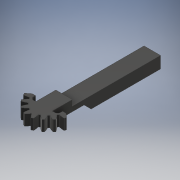
# Autodesk Inventor part: WA04
Saved by Autodesk Inventor 2017 (Build 210142000, 142)
## iProperties
Created: 2019-05-07
Part Number: WA04
Material: ABS Plastic
Document SubType Name: Modeling
Designer: Dell
Density: 1.06 g/cm^3
Appearance: Smooth - Black
Author: Dell
Autodesk Inventor part; units mm, degrees
ref_plane "YZ Plane" through (0, 0, 0) normal (1, 0, 0) x (0, 1, 0)
ref_plane "XZ Plane" through (0, 0, 0) normal (0, 1, 0) x (-1, 0, 0)
ref_plane "XY Plane" through (0, 0, 0) normal (0, 0, 1) x (1, 0, 0)
sketch "Sketch1" plane through (0, 0, 0) normal (0, 0, 1) x (1, 0, 0)
  line L0 (0, 0) -> (14, 0)
  line L1 (14, 0) -> (14, 100)
  line L2 (14, 100) -> (0, 100)
  line L3 (0, 100) -> (0, 0)
  dimension "d0" = 14
  dimension "d1" = 100
  constraints: 8 end point, 2 parallel, 1 horizontal, 1 perpendicular
  measures "d0" distance of L2.end L1.end
  measures "d1" distance of L1.end L0.end
extrude "Extrusion1" add sketch "Sketch1" along normal blind 10
sketch "Sketch2" plane through (0, 0, 10) normal (0, 0, 1) x (1, 0, 0)
  arc A0 (-7.2229, 7.2229) -> (-10.9281, 4.2365) centre (2.4249, -8.5384) ccw
  arc A1 (-10.9281, 4.2365) -> (-10.2545, 2.6798) centre (14.1758, 14.1758) ccw
  arc A2 (-10.2545, 2.6798) -> (-5.5411, 3.3364) centre (-10.4262, 21.1587) ccw
  arc A3 (-5.5411, 3.3364) -> (-4.8216, 2.1197) centre (14.1758, 14.1758) ccw
  arc A4 (-4.8216, 2.1197) -> (-7.6676, -1.6944) centre (8.4429, -10.7471) ccw
  arc A5 (-7.6676, -1.6944) -> (-6.628, -3.0346) centre (14.1758, 14.1758) ccw
  arc A6 (-6.628, -3.0346) -> (-2.226, -1.2265) centre (-11.3898, 14.8211) ccw
  arc A7 (-2.226, -1.2265) -> (-1.2265, -2.226) centre (14.1758, 14.1758) ccw
  arc A8 (-1.2265, -2.226) -> (-3.0346, -6.628) centre (14.8211, -11.3898) ccw
  arc A9 (-3.0346, -6.628) -> (-1.6944, -7.6676) centre (14.1758, 14.1758) ccw
  arc A10 (-1.6944, -7.6676) -> (2.1197, -4.8216) centre (-10.7471, 8.4429) ccw
  arc A11 (2.1197, -4.8216) -> (3.3364, -5.5411) centre (14.1758, 14.1758) ccw
  arc A12 (3.3364, -5.5411) -> (2.6798, -10.2545) centre (21.1587, -10.4262) ccw
  arc A13 (2.6798, -10.2545) -> (4.2365, -10.9281) centre (14.1758, 14.1758) ccw
  arc A14 (4.2365, -10.9281) -> (7.2229, -7.2229) centre (-8.5384, 2.4249) ccw
  circle A15 centre (14.1758, 14.1758) radius 22.5 construction
  circle A16 centre (14.1758, 14.1758) radius 27 construction
  line L0 (-7.2229, 7.2229) -> (7.2229, -7.2229)
  line L1 (-10.9281, 4.2365) -> (4.2365, -10.9281) construction
  line L2 (-5.5411, 3.3364) -> (3.3364, -5.5411) construction
  line L3 (-4.8216, 2.1197) -> (2.1197, -4.8216) construction
  line L4 (-10.2545, 2.6798) -> (2.6798, -10.2545) construction
  line L5 (-7.6676, -1.6944) -> (-1.6944, -7.6676) construction
  line L6 (-6.628, -3.0346) -> (-3.0346, -6.628) construction
  line L7 (-2.226, -1.2265) -> (-1.2265, -2.226) construction
  line L8 (0, 100) -> (0, 0) projected
  point P0 (-11.0317, -23.0721)
  point P1 (-4.9473, -25.0907)
  point P2 (1.448, -25.5328)
  point P3 (-1.448, -25.5328)
  point P4 (4.9473, -25.0907)
  point P5 (11.0317, -23.0721)
  point P6 (-1.3509, -1.3509)
  dimension "d4" = 18.4797
  dimension "d5" = 18.4797
  dimension "d6" = 27
  dimension "d7" = 27
  dimension "d8" = 27
  dimension "d9" = 27
  dimension "d10" = 18.4797
  dimension "d11" = 18.4797
  dimension "d12" = 22.5
  dimension "d13" = 22.5
  dimension "d14" = 22.5
  dimension "d15" = 18.4797
  dimension "d16" = 18.4797
  dimension "d17" = 18.4797
  dimension "d18" = 18.4797
  dimension "d19" = 4.7589
  dimension "d20" = 20.4296
  dimension "d21" = 21.446
  dimension "d22" = 9.8164
  dimension "d23" = 12.5546
  dimension "d24" = 18.2919
  dimension "d25" = 8.4475
  dimension "d26" = 5.0819
  dimension "d27" = 1.4135
  dimension "d28" = 1.559
  dimension "d31" = 45
  constraints: 30 point on circle, 16 end point, 15 centre point, 6 parallel, 2 coincident, 2 midpoint, 20 other
  measures "d4" radius of A0
  measures "d5" radius of A2
  measures "d6" radius of A1
  measures "d7" radius of A5
  measures "d8" radius of A9
  measures "d9" radius of A13
  measures "d10" radius of A12
  measures "d11" radius of A14
  measures "d12" radius of A11
  measures "d13" radius of A7
  measures "d14" radius of A3
  measures "d15" radius of A4
  measures "d16" radius of A6
  measures "d17" radius of A8
  measures "d18" radius of A10
  measures "d19" distance of L2.start L4.start
  measures "d20" distance of L0.start L0.end
  measures "d21" distance of L1.start L1.end
  measures "d22" distance of L3.start L3.end
  measures "d23" distance of L2.start L2.end
  measures "d24" distance of L4.start L4.end
  measures "d25" distance of L5.start L5.end
  measures "d26" distance of L6.start L6.end
  measures "d27" distance of L7.start L7.end
  measures "d28" distance between parallel lines of L0 L2
  measures "d31" angle of L8 L0
extrude "Extrusion2" add sketch "Sketch2" against normal blind 10
ref_plane "Work Plane1" through (7, 100, 0) normal (-1, 0, 0) x (0, 0, 1)
sketch "Sketch6" plane through (0, 0, 10) normal (0, 0, 1) x (1, 0, 0)
  circle A0 centre (7, 15) radius 2.5
  line L0 (14, 100) -> (0, 100) projected
  point P0 (0, 0)
  point P1 (7, 100)
  dimension "d38" = 5
  dimension "d39" = 85
  constraints: 1 centre point, 1 midpoint, 1 vertical alignment
  measures "d38" diameter of A0
  measures "d39" distance from line of L0 A0.centre
extrude "Extrusion6" cut sketch "Sketch6" against normal blind 10
sketch "Sketch7" plane through (0, 0, 0) normal (0, 0, -1) x (-1, 0, 0)
  circle A0 centre (-7, 14) radius 2
  circle A1 centre (-7, 15) radius 2.5 projected
  point P0 (0, 0)
  dimension "d42" = 4
  dimension "d43" = 1
  constraints: 1 centre point, 1 vertical alignment
  measures "d42" diameter of A0
  measures "d43" distance of A1.centre A0.centre
extrude "Extrusion7" add sketch "Sketch7" along normal blind 2 contours A0 A1 | A1 A0 picked at (-6.9413, 13.6767) picked at (-7.0758, 12.3503)
fillet "Fillet1" radius 2 1 edges at (9, 14, -2)
sketch "Sketch9" plane through (0, 0, 10) normal (0, 0, 1) x (1, 0, 0)
  circle A0 centre (7, 15) radius 2.5 projected
  point P0 (0, 0)
extrude "Extrusion9" add sketch "Sketch9" against normal blind 10
mirror "Mirror3" about plane through (7, 100, 0) normal (-1, 0, 0) of "Extrusion2"
sketch "Sketch10" plane through (0, 0, 0) normal (0, 0, -1) x (-1, 0, 0)
  line L0 (-14, 0) -> (-7, -7) projected
  line L1 (0, 0) -> (-14, 0) projected
  line L2 (0, 0) -> (-7, -7) projected
extrude "Extrusion10" add sketch "Sketch10" against normal blind 10
sketch "Sketch11" plane through (0, 0, 0) normal (0, 0, -1) x (-1, 0, 0)
  line L0 (-17, 3) -> (-14, 3)
  line L1 (-14, 0) -> (-14, 100) projected
  line L2 (-14, 3) -> (-14, 0)
  line L3 (-21.2229, 7.2229) -> (-14, 0) projected
  line L4 (-17, 3) -> (-14, 0)
  line L5 (0, 0) -> (0, 3)
  line L6 (0, 100) -> (0, 0) projected
  line L7 (0, 3) -> (3, 3)
  line L8 (7.2229, 7.2229) -> (0, 0) projected
  line L9 (3, 3) -> (0, 0)
  dimension "d55" = 3
  constraints: 12 end point, 3 collinear, 3 point on line, 1 horizontal, 1 horizontal alignment, 1 perpendicular
  measures "d55" distance from line of L1.start L0
extrude "Extrusion11" add sketch "Sketch11" against normal blind 10
sketch "Sketch12" plane through (0, 0, 0) normal (0, 0, -1) x (-1, 0, 0)
  line L0 (-21.2229, 7.2229) -> (-18.5, 7.2229)
  line L1 (-18.5, 7.2229) -> (-18.5, 4.5)
  line L2 (-21.2229, 7.2229) -> (-17, 3) projected
  point P0 (0, 0)
  dimension "d58" = 1.5
  constraints: 4 end point, 1 horizontal, 1 point on line, 1 vertical
  measures "d58" horizontal distance of L2.end L1.end
extrude "Extrusion12" add sketch "Sketch12" against normal blind 10
mirror "Mirror4" about plane through (7, 100, 0) normal (-1, 0, 0) of "Extrusion12"
fillet "Fillet2" radius 2 2 edges at (18.5, 4.5, 5) (-4.5, 4.5, 5)
fillet "Fillet3" radius 2 2 edges at (17, 3, 5) (-3, 3, 5)
sketch "Sketch13" plane through (0, 0, 0) normal (0, 0, -1) x (-1, 0, 0)
  line L0 (-14, 3) -> (-14, 100) projected
  line L1 (0, 100) -> (0, 3) projected
  line L2 (-14, 100) -> (0, 100)
  line L3 (0, 100) -> (0, 20)
  line L4 (0, 20) -> (-14, 20)
  line L5 (-14, 20) -> (-14, 100)
  point P0 (0, 0)
  dimension "d63" = 80
  constraints: 8 end point, 2 parallel, 1 horizontal, 1 perpendicular, 1 point on line
  measures "d63" distance between parallel lines of L2 L4
extrude "Extrusion13" cut sketch "Sketch13" against normal through all
sketch "Sketch15" plane through (14, 3, 10) normal (1, 0, 0) x (0, 0, -1)
  line L0 (0, 17) -> (10, 17) projected
  line L1 (6, 17) -> (6, 92)
  line L2 (6, 92) -> (16, 92)
  line L3 (16, 92) -> (16, 27)
  line L4 (10, 17) -> (6, 17)
  line L5 (10, 0) -> (10, 17) projected
  line L6 (10, 17) -> (0, 17) projected
  line L7 (10, 17) -> (10, 27)
  line L8 (10, 27) -> (16, 27)
  point P0 (10, -3)
  dimension "d74" = 6
  dimension "d75" = 10
  dimension "d76" = 75
  dimension "d80" = 10
  constraints: 12 end point, 4 perpendicular, 2 vertical, 1 point on line
  measures "d74" distance from line of L0.start L1
  measures "d75" distance between parallel lines of L3 L1
  measures "d76" distance between parallel lines of L0 L2
  measures "d80" distance of L0.end L7.end
extrude "Extrusion15" add sketch "Sketch15" against normal blind 14
chamfer "Chamfer1" distance 6 angle 45 1 edges at (7, 30, -6)
sketch "Sketch16" plane through (0, 0, 10) normal (0, 0, 1) x (1, 0, 0)
  circle A0 centre (7, 14) radius 2 projected
  line L0 (14, 20) -> (0, 20) projected
  line L1 (0, 20) -> (0, 3) projected
  line L2 (0, 3) -> (-2.1716, 3) projected
  arc A1 (-3.5858, 3.5858) -> (-2.1716, 3) centre (-2.1716, 5) ccw projected
  line L3 (-3.9142, 3.9142) -> (-3.5858, 3.5858) projected
  arc A2 (-4.5, 5.3284) -> (-3.9142, 3.9142) centre (-2.5, 5.3284) ccw projected
  line L4 (-4.5, 7.2229) -> (-4.5, 5.3284) projected
  line L5 (-7.2229, 7.2229) -> (-4.5, 7.2229) projected
  arc A3 (-7.2229, 7.2229) -> (-10.9281, 4.2365) centre (2.4249, -8.5384) ccw projected
  arc A4 (-10.9281, 4.2365) -> (-10.2545, 2.6798) centre (14.1758, 14.1758) ccw projected
  arc A5 (-10.2545, 2.6798) -> (-5.5411, 3.3364) centre (-10.4262, 21.1587) ccw projected
  arc A6 (-5.5411, 3.3364) -> (-4.8216, 2.1197) centre (14.1758, 14.1758) ccw projected
  arc A7 (-4.8216, 2.1197) -> (-7.6676, -1.6944) centre (8.4429, -10.7471) ccw projected
  arc A8 (-7.6676, -1.6944) -> (-6.628, -3.0346) centre (14.1758, 14.1758) ccw projected
  arc A9 (-6.628, -3.0346) -> (-2.226, -1.2265) centre (-11.3898, 14.8211) ccw projected
  arc A10 (-2.226, -1.2265) -> (-1.2265, -2.226) centre (14.1758, 14.1758) ccw projected
  arc A11 (-1.2265, -2.226) -> (-3.0346, -6.628) centre (14.8211, -11.3898) ccw projected
  arc A12 (-3.0346, -6.628) -> (-1.6944, -7.6676) centre (14.1758, 14.1758) ccw projected
  arc A13 (-1.6944, -7.6676) -> (2.1197, -4.8216) centre (-10.7471, 8.4429) ccw projected
  arc A14 (2.1197, -4.8216) -> (3.3364, -5.5411) centre (14.1758, 14.1758) ccw projected
  arc A15 (3.3364, -5.5411) -> (2.6798, -10.2545) centre (21.1587, -10.4262) ccw projected
  arc A16 (2.6798, -10.2545) -> (4.2365, -10.9281) centre (14.1758, 14.1758) ccw projected
  arc A17 (4.2365, -10.9281) -> (7, -7.578) centre (-8.5384, 2.4249) ccw projected
  arc A18 (7, -7.578) -> (9.7635, -10.9281) centre (22.5384, 2.4249) ccw projected
  arc A19 (9.7635, -10.9281) -> (11.3202, -10.2545) centre (-0.1758, 14.1758) ccw projected
  arc A20 (11.3202, -10.2545) -> (10.6636, -5.5411) centre (-7.1587, -10.4262) ccw projected
  arc A21 (10.6636, -5.5411) -> (11.8803, -4.8216) centre (-0.1758, 14.1758) ccw projected
  arc A22 (11.8803, -4.8216) -> (15.6944, -7.6676) centre (24.7471, 8.4429) ccw projected
  arc A23 (15.6944, -7.6676) -> (17.0346, -6.628) centre (-0.1758, 14.1758) ccw projected
  arc A24 (17.0346, -6.628) -> (15.2265, -2.226) centre (-0.8211, -11.3898) ccw projected
  arc A25 (15.2265, -2.226) -> (16.226, -1.2265) centre (-0.1758, 14.1758) ccw projected
  arc A26 (16.226, -1.2265) -> (20.628, -3.0346) centre (25.3898, 14.8211) ccw projected
  arc A27 (20.628, -3.0346) -> (21.6676, -1.6944) centre (-0.1758, 14.1758) ccw projected
  arc A28 (21.6676, -1.6944) -> (18.8216, 2.1197) centre (5.5571, -10.7471) ccw projected
  arc A29 (18.8216, 2.1197) -> (19.5411, 3.3364) centre (-0.1758, 14.1758) ccw projected
  arc A30 (19.5411, 3.3364) -> (24.2545, 2.6798) centre (24.4262, 21.1587) ccw projected
  arc A31 (24.2545, 2.6798) -> (24.9281, 4.2365) centre (-0.1758, 14.1758) ccw projected
  arc A32 (24.9281, 4.2365) -> (21.2229, 7.2229) centre (11.5751, -8.5384) ccw projected
  line L6 (21.2229, 7.2229) -> (18.5, 7.2229) projected
  line L7 (18.5, 7.2229) -> (18.5, 5.3284) projected
  arc A33 (17.9142, 3.9142) -> (18.5, 5.3284) centre (16.5, 5.3284) ccw projected
  line L8 (17.9142, 3.9142) -> (17.5858, 3.5858) projected
  arc A34 (16.1716, 3) -> (17.5858, 3.5858) centre (16.1716, 5) ccw projected
  line L9 (16.1716, 3) -> (14, 3) projected
  line L10 (14, 3) -> (14, 20) projected
  point P0 (0, 0)
extrude "Extrusion16" cut sketch "Sketch16" against normal blind 1 contours A0 | L10 L9 A34 L8 A33 L7 L6 A32 A31 A30 A29 A28 A27 A26 A25 A24 A23 A22 A21 A20 A19 A18 A17 A16 A15 A14 A13 A12 A11 A10 A9 A8 A7 A6 A5 A4 A3 L5 L4 A2 L3 A1 L2 L1 L0
body "Solid1"
